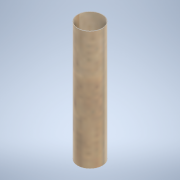
# Autodesk Inventor part: insulation
Saved by Autodesk Inventor 2021 (Build 250183000, 183)
## iProperties
Created: 2021-04-18
Part Number: insulation
Material: Wood (Maple)
Document SubType Name: Modeling
Designer: samlo
Density: 0.67 g/cm^3
Appearance: Natural Maple - Glossy Dark Tint
Author: samlo
Autodesk Inventor part; units mm, degrees
ref_plane "YZ Plane" through (0, 0, 0) normal (1, 0, 0) x (0, 1, 0)
ref_plane "XZ Plane" through (0, 0, 0) normal (0, 1, 0) x (-1, 0, 0)
ref_plane "XY Plane" through (0, 0, 0) normal (0, 0, 1) x (1, 0, 0)
sketch "Sketch1" plane through (0, 0, 0) normal (0, 0, 1) x (1, 0, 0)
  line L0 (15, 0) -> (15.5, 0)
  line L1 (15.5, 0) -> (15.5, 150)
  line L2 (15.5, 150) -> (15, 150)
  line L3 (15, 150) -> (15, 0)
  line L4 (0, -30) -> (0, 180) projected
  point P0 (0, 0)
  dimension "d0" = 15
  dimension "d1" = 15.5
  dimension "d2" = 150
  constraints: 8 end point, 2 parallel, 1 horizontal, 1 perpendicular
  measures "d0" distance of L0.start point (0, 0)
  measures "d1" distance of L0.end point (0, 0)
  measures "d2" distance of L2.end L0.start
revolve "Revolution1" add sketch "Sketch1" angle 360 about axis through (0, -10, 0) along (0, 1, 0)
body "Solid1"
